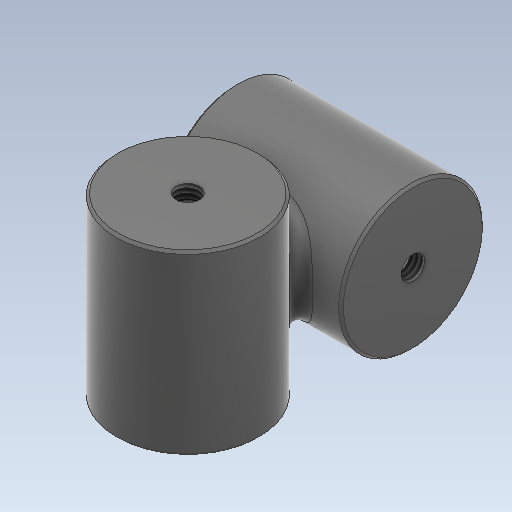
# Autodesk Inventor part: Swivel
Saved by Autodesk Inventor 2020 (Build 240168000, 168)
## iProperties
Created: 2021-07-08
Part Number: Swivel
Material: Steel, Carbon
Document SubType Name: Modeling
Designer: Simon.Alvarez
Density: 7.85 g/cm^3
Appearance: Semi-Polished
Author: Simon.Alvarez
Autodesk Inventor part; units mm, degrees
ref_plane "YZ Plane" through (0, 0, 0) normal (1, 0, 0) x (0, 1, 0)
ref_plane "XZ Plane" through (0, 0, 0) normal (0, 1, 0) x (-1, 0, 0)
ref_plane "XY Plane" through (0, 0, 0) normal (0, 0, 1) x (1, 0, 0)
sketch "Sketch1" plane through (0, 0, 0) normal (0, 1, 0) x (-1, 0, 0)
  circle A0 centre (0, 0) radius 15
  dimension "d0" = 30
  constraints: 1 centre point, 1 coincident
  measures "d0" diameter of A0
extrude "Extrusion1" add sketch "Sketch1" along normal mid plane 37
shell "Shell1" thickness 3 removed faces 0
chamfer "Chamfer1" distance 0.5 angle 45 2 edges at (15, 18.5, 0) (15, -18.5, 0)
sketch "Sketch2" plane through (0, 18.5, 0) normal (0, 1, 0) x (1, 0, 0)
  point P0 (0, 0)
  point P1 (0, 0)
  constraints: 1 coincident
hole "Hole1" at (0, 18.5, 0) direction (0, -1, 0) diameter 4.917 end through all thread size "M6x1" class "6H" standard "ANSI Metric M Profile"
sketch "Sketch4" plane through (0, 0, 0) normal (1, 0, 0) x (0, 1, 0)
  circle A0 centre (0, -28.5) radius 15
  line L0 (-21, 0) -> (21, 0) projected
  point P0 (0, 0)
  dimension "d16" = 30
  dimension "d17" = 28.5
  constraints: 1 centre point
  measures "d16" diameter of A0
  measures "d17" distance from line of L0 A0.centre
extrude "Extrusion2" add sketch "Sketch4" along normal mid plane 37
shell "Shell2" thickness 3 removed faces 0
chamfer "Chamfer2" distance 0.5 angle 45 6 edges at (18.5, 0, -13.5) (18.5, -8.5393, -40.8321) (18.5, 12.3321, -19.9607) (-18.5, 0, -13.5) (-18.5, -8.5393, -40.8321) (-18.5, 12.3321, -19.9607)
sketch "Sketch6" plane through (18.5, 0, -28.5) normal (1, 0, 0) x (0, 0, -1)
  point P0 (-28.5, 0)
  point P1 (0, 0)
hole "Hole2" at (18.5, 0, -28.5) direction (-1, 0, 0) diameter 4.917 end through all thread size "M6x1" class "6H" standard "ANSI Metric M Profile"
fillet "Fillet1" radius 2 4 edges at (4.6839, 4.6836, -14.2499) (4.6837, -4.6837, -14.25) (-4.6837, 4.6838, -14.25) (-4.6837, -4.6838, -14.25)
equation "\"d1\" = Length"
equation "\"d16\" = Dia"
equation "\"d17\" = 0.95 * Dia"
equation "\"d18\" = Length"
equation "\"Dia\" = 30"
equation "\"Length\" = 37"
body "Solid1"
